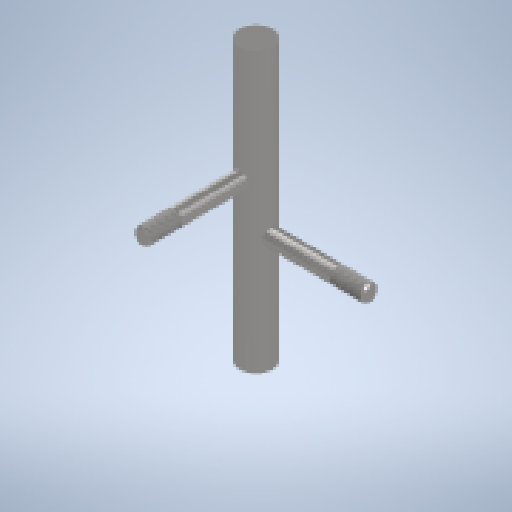
# Autodesk Inventor part: HTW-000681
Saved by Autodesk Inventor 2024.4 (Build 284460000, 460)
## iProperties
Created: 2026-01-12
Part Number: HTW-000681
Material: Edelstahl
Document SubType Name: Modeling
Designer: PC
Density: 8 g/cm^3
Appearance: Halbpoliert
Description: Steuerteil
Mass: 387.528 g
Surface Area: 187.487 cm^2
Volume: 48.441 cm^3
Masse[kg]: 0,272 kg
Autodesk Inventor part; units mm, degrees
ref_plane "YZ Plane" through (0, 0, 0) normal (1, 0, 0) x (0, 1, 0)
ref_plane "XZ Plane" through (0, 0, 0) normal (0, 1, 0) x (-1, 0, 0)
ref_plane "XY Plane" through (0, 0, 0) normal (0, 0, 1) x (1, 0, 0)
sketch "Skizze1" plane through (0, 0, 0) normal (0, 0, 1) x (1, 0, 0)
  circle A0 centre (0, 0) radius 10
  dimension "d0" = 20
  constraints: 1 centre point, 1 coincident
  measures "d0" diameter of A0
extrude "Extrusion1" add sketch "Skizze1" along normal blind 170
sketch "Skizze5" plane through (0, 0, 0) normal (0, 1, 0) x (-1, 0, 0)
  circle A0 centre (0, 100) radius 5
  line L0 (0, -21) -> (0, 126) projected
  line L1 (7, 0) -> (-7, 0) projected
  point P0 (0, 0)
  dimension "d11" = 10
  dimension "d12" = 0
  dimension "d13" = 100
  constraints: 1 centre point
  measures "d11" diameter of A0
  measures "d12" distance from line of L0 A0.centre
  measures "d13" distance from line of L1 A0.centre
extrude "Extrusion4" add sketch "Skizze5" against normal blind 70
sketch "Skizze6" plane through (0, 0, 0) normal (1, 0, 0) x (0, 1, 0)
  line L0 (10, 170) -> (-10, 170) projected
  line L1 (0, 170) -> (0, 70)
  circle A0 centre (0, 70) radius 5
  point P0 (0, 0)
  dimension "d17" = 100
  dimension "d18" = 10
  constraints: 2 end point, 1 centre point, 1 coincident, 1 midpoint, 1 vertical
  measures "d17" distance of L1.start L1.end
  measures "d18" diameter of A0
extrude "Extrusion5" add sketch "Skizze6" along normal blind 70
sketch "Skizze7" plane through (0, 0, 0) normal (0, 0, -1) x (-1, 0, 0)
  circle A0 centre (0, 0) radius 8.5
  constraints: 1 centre point, 1 coincident
extrude "Extrusion6" cut sketch "Skizze7" against normal blind 60
thread "Gewinde1" size "M10x1.5" class "6g" standard "ANSI Metric M Profile" length 20
thread "Gewinde2" size "M10x1.5" class "6g" standard "ANSI Metric M Profile" length 20
chamfer "Fasen1" distance 1 angle 45 1 edges at (5, -70, 100)
chamfer "Fasen2" distance 1 angle 45 1 edges at (70, -5, 70)
sketch "Skizze8" plane through (0, 0, 170) normal (0, 0, 1) x (1, 0, 0)
  point P0 (0, 0)
hole "Bohrung1" at (0, 0, 170) direction (0, 0, -1) diameter 6.647 depth 22.2 tip angle 118 thread size "M8x1.25" class "6H" standard "ISO Metric profile"
